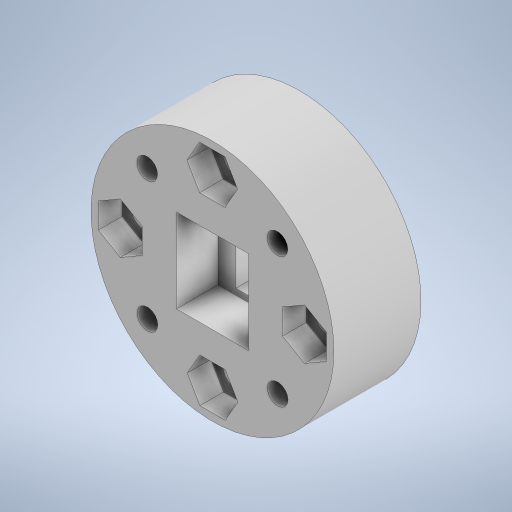
# Autodesk Inventor part: GripperBaseCircularLower
Saved by Autodesk Inventor 2023 (Build 270158000, 158)
## iProperties
Created: 2023-06-03
Part Number: GripperBaseCircularLower
Material: Ogólny
Document SubType Name: Modeling
Designer: Kamil
Density: 1 g/cm^3
Appearance: Domyślna
Author: Kamil
Autodesk Inventor part; units mm, degrees
ref_plane "YZ Plane" through (0, 0, 0) normal (1, 0, 0) x (0, 1, 0)
ref_plane "XZ Plane" through (0, 0, 0) normal (0, 1, 0) x (-1, 0, 0)
sketch "Szkic1" plane through (0, 0, 0) normal (0, 0, 1) x (1, 0, 0)
  line L0 (24.72, -24.72) -> (24.72, -14.42)
  line L1 (25.2197, -24.72) -> (24.72, -24.72)
  line L2 (24.72, -14.42) -> (25.2197, -14.42)
  line L3 (0, -39.14) -> (10.3, -39.14)
  line L4 (-14.42, -14.42) -> (-14.42, -24.72)
  line L5 (10.3, 0) -> (0, 0)
  line L6 (10.225, -25.645) -> (10.225, -13.495)
  line L7 (10.225, -25.645) -> (0.075, -25.645)
  line L8 (0.075, -13.495) -> (0.075, -25.645)
  line L9 (0.075, -13.495) -> (10.225, -13.495)
  line L10 (-14.9619, -24.72) -> (-14.9619, -24.7024)
  arc A0 (-14.9619, -24.7024) -> (0.075, -39.676) centre (5.1314, -19.5612) ccw
  arc A1 (10.3, -39.6475) -> (25.2201, -24.72) centre (5.1314, -19.5612) ccw
  line L11 (-14.9619, -14.42) -> (-14.42, -14.42)
  line L12 (24.72, -14.42) -> (25.2247, -14.42)
  line L13 (-14.42, -24.72) -> (-14.9619, -24.72)
  line L14 (0.075, -39.14) -> (0.075, -39.676)
  line L15 (0.075, 0.5536) -> (0.075, 0)
  line L16 (0.075, -13.495) -> (0.075, -25.645)
  line L17 (10.3, -39.6475) -> (10.3, -39.14)
  line L18 (10.3, 0) -> (10.3, 0.5251)
  line L19 (25.2201, -24.72) -> (24.72, -24.72)
  arc A2 (25.2247, -14.42) -> (10.3, 0.5251) centre (5.1314, -19.5612) ccw
  arc A3 (0.075, 0.5536) -> (-14.9619, -14.42) centre (5.1314, -19.5612) ccw
  circle A4 centre (5.1581, -35.1055) radius 1.75
  circle A5 centre (16.1418, -30.5337) radius 1.75
  circle A6 centre (20.6757, -19.5344) radius 1.75
  circle A7 centre (16.1039, -8.5508) radius 1.75
  circle A8 centre (5.1046, -4.0169) radius 1.75
  circle A9 centre (-5.879, -8.5887) radius 1.75
  circle A10 centre (-10.4129, -19.588) radius 1.75
  circle A11 centre (-5.8412, -30.5716) radius 1.75
  point P0 (5.15, -19.57)
  point P1 (-14.9574, -24.72)
  dimension "d0" = 3.5
  dimension "d3" = 360
  constraints: 40 end point, 12 centre point, 10 parallel, 8 point on circle, 2 horizontal, 2 point on line, 1 coincident, 17 other
  measures "d0" diameter of A4
extrude "Wyciągnięcie proste1" add sketch "Szkic1" along normal blind 9.7 contours L1 A1 L17 L3 L14 A0 L13 L4 L11 A3 L15 L5 L18 A2 L12 L2 L0
sketch "Szkic2" plane through (0, 0, 0) normal (0, 0, -1) x (-1, 0, 0)
  circle A0 centre (-16.1039, -8.5508) radius 1.75 projected
  circle A1 centre (-16.1039, -8.5508) radius 2.9
  arc A2 (-10.3, 0.5251) -> (-25.2247, -14.42) centre (-5.1314, -19.5612) ccw projected
  arc A3 (-0.075, -39.676) -> (14.9574, -24.72) centre (-5.1314, -19.5612) ccw projected
  circle A4 centre (-16.1418, -30.5337) radius 2.9
  circle A5 centre (5.8412, -30.5716) radius 2.9
  circle A6 centre (5.879, -8.5887) radius 2.9
  line L0 (-13.226, -10.2628) -> (-16.1476, -11.8991)
  line L1 (-16.1476, -11.8991) -> (-19.0255, -10.1871)
  line L2 (-19.0255, -10.1871) -> (-18.9818, -6.8387)
  line L3 (-18.9818, -6.8387) -> (-16.0602, -5.2024)
  line L4 (-16.0602, -5.2024) -> (-13.1823, -6.9145)
  line L5 (-13.1823, -6.9145) -> (-13.226, -10.2628)
  line L6 (-19.7668, -16.3115) -> (-17.4301, -18.71)
  line L7 (-23.0124, -17.1359) -> (-19.7668, -16.3115)
  line L8 (-23.9212, -20.3588) -> (-23.0124, -17.1359)
  line L9 (-21.5845, -22.7574) -> (-23.9212, -20.3588)
  line L10 (-18.3389, -21.933) -> (-21.5845, -22.7574)
  line L11 (-17.4301, -18.71) -> (-18.3389, -21.933)
  line L12 (-17.7781, -27.6121) -> (-14.4297, -27.6559)
  line L13 (-19.4901, -30.49) -> (-17.7781, -27.6121)
  line L14 (-17.8538, -33.4116) -> (-19.4901, -30.49)
  line L15 (-14.5055, -33.4554) -> (-17.8538, -33.4116)
  line L16 (-12.7934, -30.5775) -> (-14.5055, -33.4554)
  line L17 (-14.4297, -27.6559) -> (-12.7934, -30.5775)
  line L18 (-8.3811, -34.1966) -> (-5.9825, -31.8599)
  line L19 (-7.5567, -37.4422) -> (-8.3811, -34.1966)
  line L20 (-4.3338, -38.3511) -> (-7.5567, -37.4422)
  line L21 (-1.9352, -36.0143) -> (-4.3338, -38.3511)
  line L22 (-2.7596, -32.7688) -> (-1.9352, -36.0143)
  line L23 (-5.9825, -31.8599) -> (-2.7596, -32.7688)
  line L24 (2.9196, -32.2079) -> (2.9633, -28.8596)
  line L25 (5.7974, -33.92) -> (2.9196, -32.2079)
  line L26 (8.7191, -32.2837) -> (5.7974, -33.92)
  line L27 (8.7628, -28.9353) -> (8.7191, -32.2837)
  line L28 (5.8849, -27.2233) -> (8.7628, -28.9353)
  line L29 (2.9633, -28.8596) -> (5.8849, -27.2233)
  line L30 (9.5041, -22.8109) -> (7.1674, -20.4124)
  line L31 (12.7496, -21.9865) -> (9.5041, -22.8109)
  line L32 (13.6585, -18.7636) -> (12.7496, -21.9865)
  line L33 (11.3218, -16.365) -> (13.6585, -18.7636)
  line L34 (8.0762, -17.1894) -> (11.3218, -16.365)
  line L35 (7.1674, -20.4124) -> (8.0762, -17.1894)
  line L36 (7.5153, -11.5103) -> (4.167, -11.4666)
  line L37 (9.2274, -8.6324) -> (7.5153, -11.5103)
  line L38 (7.5911, -5.7108) -> (9.2274, -8.6324)
  line L39 (4.2427, -5.667) -> (7.5911, -5.7108)
  line L40 (2.5307, -8.5449) -> (4.2427, -5.667)
  line L41 (4.167, -11.4666) -> (2.5307, -8.5449)
  line L42 (-1.8817, -4.9258) -> (-4.2802, -7.2625)
  line L43 (-2.706, -1.6802) -> (-1.8817, -4.9258)
  line L44 (-5.929, -0.7713) -> (-2.706, -1.6802)
  line L45 (-8.3275, -3.1081) -> (-5.929, -0.7713)
  line L46 (-7.5031, -6.3536) -> (-8.3275, -3.1081)
  line L47 (-4.2802, -7.2625) -> (-7.5031, -6.3536)
  point P0 (0, 0)
  point P1 (-13.2042, -8.5887)
  point P2 (-18.5984, -17.5108)
  point P3 (-16.1039, -27.634)
  point P4 (-7.1818, -33.0283)
  point P5 (2.9414, -30.5337)
  point P6 (8.3357, -21.6116)
  point P7 (5.8412, -11.4884)
  point P8 (-3.0809, -6.0941)
  dimension "d7" = 5.8
  dimension "d10" = 360
  dimension "d22" = 360
  constraints: 96 end point, 3 centre point, 2 coincident, 1 midpoint, 130 other
extrude "Wyciągnięcie proste2" cut sketch "Szkic2" against normal blind 3.7 contours A1 | A4 | A5 | A6
sketch "Szkic3" plane through (0, 0, 0) normal (0, 0, -1) x (-1, 0, 0)
  circle A0 centre (5.8412, -30.5716) radius 2.9 projected
  circle A1 centre (5.879, -8.5887) radius 2.9 projected
  circle A2 centre (-16.1418, -30.5337) radius 2.9 projected
  circle A3 centre (-16.1039, -8.5508) radius 2.9 projected
  line L0 (-24.72, -14.42) -> (-25.2247, -14.42) projected
  line L1 (-24.72, -24.72) -> (-24.72, -14.42) projected
  line L2 (-25.2201, -24.72) -> (-24.72, -24.72) projected
  arc A4 (-25.2201, -24.72) -> (-10.3, -39.6475) centre (-5.1314, -19.5612) ccw projected
  line L3 (-10.3, -39.14) -> (-10.3, -39.6475) projected
  line L4 (-0.075, -39.14) -> (-10.3, -39.14) projected
  line L5 (-0.075, -39.676) -> (-0.075, -39.14) projected
  arc A5 (-0.075, -39.676) -> (14.9574, -24.72) centre (-5.1314, -19.5612) ccw projected
  line L6 (14.42, -24.72) -> (14.9574, -24.72) projected
  line L7 (14.42, -14.42) -> (14.42, -24.72) projected
  line L8 (14.9619, -14.42) -> (14.42, -14.42) projected
  arc A6 (14.9619, -14.42) -> (-0.075, 0.5536) centre (-5.1314, -19.5612) ccw projected
  line L9 (-0.075, 0) -> (-0.075, 0.5536) projected
  line L10 (-10.3, 0) -> (-0.075, 0) projected
  line L11 (-10.3, 0.5251) -> (-10.3, 0) projected
  arc A7 (-10.3, 0.5251) -> (-25.2247, -14.42) centre (-5.1314, -19.5612) ccw projected
  circle A8 centre (10.4129, -19.588) radius 1.75 projected
  circle A9 centre (-5.1581, -35.1055) radius 1.75 projected
  circle A10 centre (-20.6757, -19.5344) radius 1.75 projected
  circle A11 centre (-5.1046, -4.0169) radius 1.75 projected
  line L12 (-10.225, -25.645) -> (-0.075, -25.645) projected
  line L13 (-10.225, -13.495) -> (-10.225, -25.645) projected
  line L14 (-0.075, -13.495) -> (-10.225, -13.495) projected
  line L15 (-0.075, -25.645) -> (-0.075, -13.495) projected
  line L16 (-10.225, -13.495) -> (-8.225, -13.495)
  line L17 (-8.225, -13.495) -> (-8.225, -25.645)
  line L18 (-8.225, -25.645) -> (-10.225, -25.645)
  line L19 (-10.225, -25.645) -> (-10.225, -13.495)
  line L20 (-0.075, -25.645) -> (-2.075, -25.645)
  line L21 (-2.075, -25.645) -> (-2.075, -13.495)
  line L22 (-2.075, -13.495) -> (-0.075, -13.495)
  line L23 (-0.075, -13.495) -> (-0.075, -25.645)
  point P0 (0, 0)
  dimension "d14" = 2
  dimension "d15" = 2
  constraints: 16 end point, 4 parallel, 2 horizontal, 2 perpendicular, 2 point on line
  measures "d14" distance of L17.end L18.end
  measures "d15" distance of L21.end L22.end
extrude "Wyciągnięcie proste3" add sketch "Szkic3" against normal blind 4.7 contours L13 L14 L17 L12 | L21 L14 L15 L12
sketch "Szkic4" plane through (0, 0, 9.7) normal (0, 0, 1) x (1, 0, 0)
  line L0 (24.72, -14.42) -> (25.2247, -14.42) projected
  arc A0 (25.2247, -14.42) -> (10.3, 0.5251) centre (5.1314, -19.5612) ccw projected
  line L1 (10.3, 0.5251) -> (10.3, 0) projected
  line L2 (10.3, 0) -> (0.075, 0) projected
  line L3 (0.075, 0) -> (0.075, 0.5536) projected
  arc A1 (0.075, 0.5536) -> (-14.9619, -14.42) centre (5.1314, -19.5612) ccw projected
  line L4 (-14.9619, -14.42) -> (-14.42, -14.42) projected
  line L5 (-14.42, -14.42) -> (-14.42, -24.72) projected
  line L6 (-14.42, -24.72) -> (-14.9574, -24.72) projected
  arc A2 (-14.9574, -24.72) -> (0.075, -39.676) centre (5.1314, -19.5612) ccw projected
  line L7 (0.075, -39.676) -> (0.075, -39.14) projected
  line L8 (0.075, -39.14) -> (10.3, -39.14) projected
  line L9 (10.3, -39.14) -> (10.3, -39.6475) projected
  arc A3 (10.3, -39.6475) -> (25.2201, -24.72) centre (5.1314, -19.5612) ccw projected
  line L10 (25.2201, -24.72) -> (24.72, -24.72) projected
  line L11 (24.72, -24.72) -> (24.72, -14.42) projected
  circle A4 centre (-10.4129, -19.588) radius 1.75 projected
  circle A5 centre (5.1581, -35.1055) radius 1.75 projected
  circle A6 centre (20.6757, -19.5344) radius 1.75 projected
  circle A7 centre (5.1046, -4.0169) radius 1.75 projected
  circle A8 centre (-5.8412, -30.5716) radius 1.75 projected
  circle A9 centre (-5.879, -8.5887) radius 1.75 projected
  circle A10 centre (16.1039, -8.5508) radius 1.75 projected
  circle A11 centre (16.1418, -30.5337) radius 1.75 projected
  line L12 (10.225, -25.645) -> (0.075, -25.645) projected
  line L13 (0.075, -25.645) -> (0.075, -13.495) projected
  line L14 (0.075, -13.495) -> (10.225, -13.495) projected
  line L15 (10.225, -13.495) -> (10.225, -25.645) projected
  line L16 (10.3, 0.5251) -> (10.3, 0) projected
  line L17 (10.3, 0.5251) -> (0.075, 0.5536)
  line L18 (10.3, 0) -> (0.075, 0) projected
  circle A12 centre (5.1314, -19.5612) radius 20.2325
  point P0 (0, 0)
  point P1 (-14.4371, -14.42)
  point P2 (0.075, 0.0293)
  point P3 (0.075, -39.1517)
  point P4 (-14.4324, -24.72)
  point P5 (24.72, -24.6249)
  point P6 (10.2329, -39.14)
  point P7 (24.72, -14.4975)
  constraints: 2 end point, 1 coincident, 3 other
extrude "Wyciągnięcie proste4" cut sketch "Szkic4" against normal through all contours L11 A12 L1 A0 L0 | L11 L10 A3 L9 L8 A12 | L7 A2 L6 A12 | A12 L4 A1 L3
sketch "Szkic5" plane through (0, 0, 0) normal (0, 0, -1) x (-1, 0, 0)
  circle A0 centre (-16.1039, -8.5508) radius 2.9 projected
  circle A1 centre (-16.1039, -8.5508) radius 2.9 projected
  line L0 (-13.2039, -10.2251) -> (-16.1039, -11.8994)
  line L1 (-16.1039, -11.8994) -> (-19.0039, -10.2251)
  line L2 (-19.0039, -10.2251) -> (-19.0039, -6.8765)
  line L3 (-19.0039, -6.8765) -> (-16.1039, -5.2022)
  line L4 (-16.1039, -5.2022) -> (-13.2039, -6.8765)
  line L5 (-13.2039, -6.8765) -> (-13.2039, -10.2251)
  arc A2 (-10.3, 0) -> (-24.72, -14.4975) centre (-5.1314, -19.5612) ccw projected
  line L6 (-17.4411, -18.6677) -> (-18.3078, -21.9023)
  line L7 (-18.3078, -21.9023) -> (-21.5423, -22.769)
  line L8 (-21.5423, -22.769) -> (-23.9102, -20.4011)
  line L9 (-23.9102, -20.4011) -> (-23.0435, -17.1666)
  line L10 (-23.0435, -17.1666) -> (-19.809, -16.2999)
  line L11 (-19.809, -16.2999) -> (-17.4411, -18.6677)
  line L12 (-14.4675, -27.6337) -> (-12.7931, -30.5337)
  line L13 (-12.7931, -30.5337) -> (-14.4675, -33.4337)
  line L14 (-14.4675, -33.4337) -> (-17.8161, -33.4337)
  line L15 (-17.8161, -33.4337) -> (-19.4904, -30.5337)
  line L16 (-19.4904, -30.5337) -> (-17.8161, -27.6337)
  line L17 (-17.8161, -27.6337) -> (-14.4675, -27.6337)
  line L18 (-6.0248, -31.871) -> (-2.7903, -32.7377)
  line L19 (-2.7903, -32.7377) -> (-1.9236, -35.9722)
  line L20 (-1.9236, -35.9722) -> (-4.2915, -38.34)
  line L21 (-4.2915, -38.34) -> (-7.526, -37.4733)
  line L22 (-7.526, -37.4733) -> (-8.3927, -34.2388)
  line L23 (-8.3927, -34.2388) -> (-6.0248, -31.871)
  line L24 (2.9412, -28.8973) -> (5.8412, -27.223)
  line L25 (5.8412, -27.223) -> (8.7412, -28.8973)
  line L26 (8.7412, -28.8973) -> (8.7412, -32.2459)
  line L27 (8.7412, -32.2459) -> (5.8412, -33.9202)
  line L28 (5.8412, -33.9202) -> (2.9412, -32.2459)
  line L29 (2.9412, -32.2459) -> (2.9412, -28.8973)
  line L30 (7.1784, -20.4547) -> (8.0451, -17.2201)
  line L31 (8.0451, -17.2201) -> (11.2796, -16.3534)
  line L32 (11.2796, -16.3534) -> (13.6475, -18.7213)
  line L33 (13.6475, -18.7213) -> (12.7808, -21.9558)
  line L34 (12.7808, -21.9558) -> (9.5462, -22.8225)
  line L35 (9.5462, -22.8225) -> (7.1784, -20.4547)
  line L36 (4.2047, -11.4887) -> (2.5304, -8.5887)
  line L37 (2.5304, -8.5887) -> (4.2047, -5.6887)
  line L38 (4.2047, -5.6887) -> (7.5534, -5.6887)
  line L39 (7.5534, -5.6887) -> (9.2277, -8.5887)
  line L40 (9.2277, -8.5887) -> (7.5534, -11.4887)
  line L41 (7.5534, -11.4887) -> (4.2047, -11.4887)
  line L42 (-4.2379, -7.2514) -> (-7.4724, -6.3847)
  line L43 (-7.4724, -6.3847) -> (-8.3391, -3.1502)
  line L44 (-8.3391, -3.1502) -> (-5.9713, -0.7824)
  line L45 (-5.9713, -0.7824) -> (-2.7367, -1.6491)
  line L46 (-2.7367, -1.6491) -> (-1.8701, -4.8836)
  line L47 (-1.8701, -4.8836) -> (-4.2379, -7.2514)
  point P0 (0, 0)
  point P1 (-13.2039, -8.5508)
  point P2 (-20.6757, -19.5344)
  point P3 (-18.625, -17.4838)
  point P4 (-16.1418, -30.5337)
  point P5 (-16.1418, -27.6337)
  point P6 (-5.1581, -35.1055)
  point P7 (-7.2088, -33.0549)
  point P8 (5.8412, -30.5716)
  point P9 (2.9412, -30.5716)
  point P10 (10.4129, -19.588)
  point P11 (8.3623, -21.6386)
  point P12 (5.879, -8.5887)
  point P13 (5.879, -11.4887)
  point P14 (-5.1046, -4.0169)
  point P15 (-3.054, -6.0675)
  dimension "d26" = 360
  constraints: 96 end point, 1 coincident, 1 horizontal alignment, 1 midpoint, 127 other
extrude "Wyciągnięcie proste5" cut sketch "Szkic5" against normal blind 4 contours A0 | L5 L0 A0 | A0 L4 L5 | A0 L3 L4 | L0 L1 A0 | A0 L2 L3 | L1 L2 A0 | L12 L13 L14 L15 L16 L17 | L24 L25 L26 L27 L28 L29 | L36 L37 L38 L39 L40 L41
sketch "Szkic6" plane through (0, 0, 9.7) normal (0, 0, 1) x (1, 0, 0)
  line L0 (10.225, -25.645) -> (0.075, -25.645) projected
  line L1 (0.075, -25.645) -> (0.075, -13.495) projected
  line L2 (0.075, -13.495) -> (10.225, -13.495) projected
  line L3 (10.225, -13.495) -> (10.225, -25.645) projected
  circle A0 centre (16.1418, -30.5337) radius 1.75 projected
  circle A1 centre (16.1039, -8.5508) radius 1.75 projected
  circle A2 centre (-5.879, -8.5887) radius 1.75 projected
  circle A3 centre (-5.8412, -30.5716) radius 1.75 projected
  circle A4 centre (5.1046, -4.0169) radius 1.75 projected
  circle A5 centre (20.6757, -19.5344) radius 1.75 projected
  circle A6 centre (5.1581, -35.1055) radius 1.75 projected
  circle A7 centre (-10.4129, -19.588) radius 1.75 projected
  arc A8 (-14.4324, -24.72) -> (0.075, -39.1517) centre (5.1314, -19.5612) ccw projected
  line L4 (0.075, -39.1517) -> (0.075, -39.14) projected
  line L5 (0.075, -39.14) -> (10.2329, -39.14) projected
  arc A9 (10.2329, -39.14) -> (24.72, -24.6249) centre (5.1314, -19.5612) ccw projected
  line L6 (24.72, -24.6249) -> (24.72, -14.4975) projected
  arc A10 (24.72, -14.4975) -> (10.3, 0) centre (5.1314, -19.5612) ccw projected
  line L7 (10.3, 0) -> (0.075, 0) projected
  line L8 (0.075, 0) -> (0.075, 0.0293) projected
  arc A11 (0.075, 0.0293) -> (-14.4371, -14.42) centre (5.1314, -19.5612) ccw projected
  line L9 (-14.4371, -14.42) -> (-14.42, -14.42) projected
  line L10 (-14.42, -14.42) -> (-14.42, -24.72) projected
  line L11 (-14.42, -24.72) -> (-14.4324, -24.72) projected
  circle A12 centre (5.1046, -4.0169) radius 1.75 projected
  circle A13 centre (5.1046, -4.0169) radius 2.25
  circle A14 centre (-10.4129, -19.588) radius 1.75 projected
  circle A15 centre (-10.4129, -19.588) radius 2.25
  circle A16 centre (5.1581, -35.1055) radius 1.75 projected
  circle A17 centre (5.1581, -35.1055) radius 2.25
  circle A18 centre (20.6757, -19.5344) radius 2.25
  point P0 (0, 0)
  dimension "d30" = 4.5
  dimension "d31" = 4.5
  dimension "d32" = 4.5
  dimension "d33" = 4.5
  constraints: 4 centre point, 4 coincident
  measures "d30" diameter of A13
  measures "d31" diameter of A15
  measures "d32" diameter of A17
  measures "d33" diameter of A18
extrude "Wyciągnięcie proste6" cut sketch "Szkic6" against normal through all contours A4 | A5 | A6 | A7 | A13 | A15 | A17 | A18
sketch "Szkic7" plane through (0, 0, 9.7) normal (0, 0, 1) x (1, 0, 0)
  circle A0 centre (5.1581, -35.1055) radius 2.25 projected
  circle A1 centre (-10.4129, -19.588) radius 2.25 projected
  circle A2 centre (20.6757, -19.5344) radius 2.25 projected
  circle A3 centre (5.1046, -4.0169) radius 2.25 projected
  line L0 (10.225, -25.645) -> (0.075, -25.645) projected
  line L1 (0.075, -25.645) -> (0.075, -13.495) projected
  line L2 (0.075, -13.495) -> (10.225, -13.495) projected
  line L3 (10.225, -13.495) -> (10.225, -25.645) projected
  circle A4 centre (16.1418, -30.5337) radius 1.75 projected
  circle A5 centre (16.1039, -8.5508) radius 1.75 projected
  circle A6 centre (-5.879, -8.5887) radius 1.75 projected
  circle A7 centre (-5.8412, -30.5716) radius 1.75 projected
  arc A8 (-14.4324, -24.72) -> (0.075, -39.1517) centre (5.1314, -19.5612) ccw projected
  line L4 (0.075, -39.1517) -> (0.075, -39.14) projected
  line L5 (0.075, -39.14) -> (10.2329, -39.14) projected
  arc A9 (10.2329, -39.14) -> (24.72, -24.6249) centre (5.1314, -19.5612) ccw projected
  line L6 (24.72, -24.6249) -> (24.72, -14.4975) projected
  arc A10 (24.72, -14.4975) -> (10.3, 0) centre (5.1314, -19.5612) ccw projected
  line L7 (10.3, 0) -> (0.075, 0) projected
  line L8 (0.075, 0) -> (0.075, 0.0293) projected
  arc A11 (0.075, 0.0293) -> (-14.4371, -14.42) centre (5.1314, -19.5612) ccw projected
  line L9 (-14.4371, -14.42) -> (-14.42, -14.42) projected
  line L10 (-14.42, -14.42) -> (-14.42, -24.72) projected
  line L11 (-14.42, -24.72) -> (-14.4324, -24.72) projected
  line L12 (-14.2545, -13.7696) -> (-14.6283, -14.1018)
  circle A12 centre (5.1314, -19.5612) radius 20.5
  point P0 (0, 0)
  dimension "d46" = 41
  dimension "d36" = 0.5
  constraints: 2 end point, 1 coincident, 1 point on circle, 3 other
  measures "d36" distance of L12.start L12.end
extrude "Wyciągnięcie proste7" add sketch "Szkic7" against normal up to surface (9.7 mm away) contours A12
sketch "Szkic8" plane through (5.1314, -19.5612, 9.7) normal (0, 0, 1) x (1, 0, 0)
  circle A0 centre (0, 0) radius 20.5 projected
  circle A1 centre (0.0268, -15.5443) radius 2.25 projected
  circle A2 centre (-15.5443, -0.0268) radius 2.25 projected
  circle A3 centre (15.5443, 0.0268) radius 2.25 projected
  circle A4 centre (-0.0268, 15.5443) radius 2.25 projected
  line L0 (5.0936, -6.0838) -> (-5.0564, -6.0838) projected
  line L1 (-5.0564, -6.0838) -> (-5.0564, 6.0662) projected
  line L2 (-5.0564, 6.0662) -> (5.0936, 6.0662) projected
  line L3 (5.0936, 6.0662) -> (5.0936, -6.0838) projected
  circle A5 centre (11.0104, -10.9725) radius 1.75 projected
  circle A6 centre (10.9725, 11.0104) radius 1.75 projected
  circle A7 centre (-11.0104, 10.9725) radius 1.75 projected
  circle A8 centre (-10.9725, -11.0104) radius 1.75 projected
  circle A9 centre (-0.0268, 15.5443) radius 3.7
  circle A10 centre (-0.0268, 15.5443) radius 2.25 projected
  line L4 (2.1094, 19.2443) -> (4.2456, 15.5443)
  line L5 (4.2456, 15.5443) -> (2.1094, 11.8443)
  line L6 (2.1094, 11.8443) -> (-2.163, 11.8443)
  line L7 (-2.163, 11.8443) -> (-4.2992, 15.5443)
  line L8 (-4.2992, 15.5443) -> (-2.163, 19.2443)
  line L9 (-2.163, 19.2443) -> (2.1094, 19.2443)
  line L10 (-6.8836, 9.8668) -> (-9.9046, 6.8457)
  line L11 (-7.9894, 13.9936) -> (-6.8836, 9.8668)
  line L12 (-9.9046, 6.8457) -> (-14.0314, 7.9515)
  line L13 (-12.1162, 15.0994) -> (-7.9894, 13.9936)
  line L14 (-15.1372, 12.0783) -> (-12.1162, 15.0994)
  circle A11 centre (-11.0104, 10.9725) radius 3.7
  line L15 (-14.0314, 7.9515) -> (-15.1372, 12.0783)
  line L16 (-11.8443, 2.1094) -> (-11.8443, -2.163)
  line L17 (-15.5443, 4.2456) -> (-11.8443, 2.1094)
  line L18 (-11.8443, -2.163) -> (-15.5443, -4.2992)
  line L19 (-19.2443, 2.1094) -> (-15.5443, 4.2456)
  line L20 (-19.2443, -2.163) -> (-19.2443, 2.1094)
  circle A12 centre (-15.5443, -0.0268) radius 3.7
  line L21 (-15.5443, -4.2992) -> (-19.2443, -2.163)
  line L22 (-9.8668, -6.8836) -> (-6.8457, -9.9046)
  line L23 (-13.9936, -7.9894) -> (-9.8668, -6.8836)
  line L24 (-6.8457, -9.9046) -> (-7.9515, -14.0314)
  line L25 (-15.0994, -12.1162) -> (-13.9936, -7.9894)
  line L26 (-12.0783, -15.1372) -> (-15.0994, -12.1162)
  circle A13 centre (-10.9725, -11.0104) radius 3.7
  line L27 (-7.9515, -14.0314) -> (-12.0783, -15.1372)
  line L28 (-2.1094, -11.8443) -> (2.163, -11.8443)
  line L29 (-4.2456, -15.5443) -> (-2.1094, -11.8443)
  line L30 (2.163, -11.8443) -> (4.2992, -15.5443)
  line L31 (-2.1094, -19.2443) -> (-4.2456, -15.5443)
  line L32 (2.163, -19.2443) -> (-2.1094, -19.2443)
  circle A14 centre (0.0268, -15.5443) radius 3.7
  line L33 (4.2992, -15.5443) -> (2.163, -19.2443)
  line L34 (6.8836, -9.8668) -> (9.9046, -6.8457)
  line L35 (7.9894, -13.9936) -> (6.8836, -9.8668)
  line L36 (9.9046, -6.8457) -> (14.0314, -7.9515)
  line L37 (12.1162, -15.0994) -> (7.9894, -13.9936)
  line L38 (15.1372, -12.0783) -> (12.1162, -15.0994)
  circle A15 centre (11.0104, -10.9725) radius 3.7
  line L39 (14.0314, -7.9515) -> (15.1372, -12.0783)
  line L40 (11.8443, -2.1094) -> (11.8443, 2.163)
  line L41 (15.5443, -4.2456) -> (11.8443, -2.1094)
  line L42 (11.8443, 2.163) -> (15.5443, 4.2992)
  line L43 (19.2443, -2.1094) -> (15.5443, -4.2456)
  line L44 (19.2443, 2.163) -> (19.2443, -2.1094)
  circle A16 centre (15.5443, 0.0268) radius 3.7
  line L45 (15.5443, 4.2992) -> (19.2443, 2.163)
  line L46 (9.8668, 6.8836) -> (6.8457, 9.9046)
  line L47 (13.9936, 7.9894) -> (9.8668, 6.8836)
  line L48 (6.8457, 9.9046) -> (7.9515, 14.0314)
  line L49 (15.0994, 12.1162) -> (13.9936, 7.9894)
  line L50 (12.0783, 15.1372) -> (15.0994, 12.1162)
  circle A17 centre (10.9725, 11.0104) radius 3.7
  line L51 (7.9515, 14.0314) -> (12.0783, 15.1372)
  point P0 (-5.1314, 19.5612)
  point P1 (-0.0268, 19.2443)
  point P2 (-13.6267, 13.5888)
  point P3 (-19.2443, -0.0268)
  point P4 (-13.5888, -13.6267)
  point P5 (0.0268, -19.2443)
  point P6 (13.6267, -13.5888)
  point P7 (19.2443, 0.0268)
  point P8 (13.5888, 13.6267)
  dimension "d39" = 7.4
  dimension "d42" = 360
  constraints: 96 end point, 2 coincident, 2 horizontal alignment, 2 vertical alignment, 1 midpoint, 162 other
extrude "Wyciągnięcie proste8" cut sketch "Szkic8" against normal blind 4 contours A1 | A2 | A3 | A4 | A9 | A9 L4 L5 | A9 L9 L4 | L5 L6 A9 | A9 L8 L9 | L6 L7 A9 | A9 L7 L8 | L16 A12 L17 | A12 | L16 L18 A12 | A12 L19 L17 | L18 L21 A12 | A12 L20 L19 | L21 L20 A12 | L28 A14 L29 | L28 L30 A14 | A14 | A14 L31 L29 | L30 L33 A14 | A14 L32 L31 | A14 L33 L32 | L40 A16 L41 | L40 L42 A16 | A16 | A16 L43 L41 | L42 L45 A16 | A16 L44 L43 | L45 L44 A16
ref_plane "Płaszczyzna konstrukcyjna1" through (0, 0, 4.85) normal (0, 0, -1) x (-1, 0, 0)
sketch "Szkic9" plane through (5.1314, -19.5612, 0) normal (0, 0, -1) x (-1, 0, 0)
  circle A0 centre (0, 0) radius 20.5 projected
  circle A1 centre (-0.0268, -15.5443) radius 2.25 projected
  circle A2 centre (15.5443, -0.0268) radius 2.25 projected
  circle A3 centre (-15.5443, 0.0268) radius 2.25 projected
  circle A4 centre (0.0268, 15.5443) radius 2.25 projected
  line L0 (10.9725, -14.359) -> (8.0725, -12.6847) projected
  line L1 (8.0725, -12.6847) -> (8.0725, -9.3361) projected
  line L2 (8.0725, -9.3361) -> (10.9725, -7.6618) projected
  line L3 (10.9725, -7.6618) -> (13.8725, -9.3361) projected
  line L4 (13.8725, -9.3361) -> (13.8725, -12.6847) projected
  line L5 (13.8725, -12.6847) -> (10.9725, -14.359) projected
  line L6 (14.359, 10.9725) -> (12.6847, 8.0725) projected
  line L7 (12.6847, 8.0725) -> (9.3361, 8.0725) projected
  line L8 (9.3361, 8.0725) -> (7.6618, 10.9725) projected
  line L9 (7.6618, 10.9725) -> (9.3361, 13.8725) projected
  line L10 (9.3361, 13.8725) -> (12.6847, 13.8725) projected
  line L11 (12.6847, 13.8725) -> (14.359, 10.9725) projected
  line L12 (-14.359, -10.9725) -> (-12.6847, -8.0725) projected
  line L13 (-12.6847, -8.0725) -> (-9.3361, -8.0725) projected
  line L14 (-9.3361, -8.0725) -> (-7.6618, -10.9725) projected
  line L15 (-7.6618, -10.9725) -> (-9.3361, -13.8725) projected
  line L16 (-9.3361, -13.8725) -> (-12.6847, -13.8725) projected
  line L17 (-12.6847, -13.8725) -> (-14.359, -10.9725) projected
  line L18 (-10.9725, 14.359) -> (-8.0725, 12.6847) projected
  line L19 (-8.0725, 12.6847) -> (-8.0725, 9.3361) projected
  line L20 (-8.0725, 9.3361) -> (-10.9725, 7.6618) projected
  line L21 (-10.9725, 7.6618) -> (-13.8725, 9.3361) projected
  line L22 (-13.8725, 9.3361) -> (-13.8725, 12.6847) projected
  line L23 (-13.8725, 12.6847) -> (-10.9725, 14.359) projected
  line L24 (-3.0936, -6.0838) -> (-3.0936, 6.0662) projected
  line L25 (3.0564, 6.0662) -> (-3.0936, 6.0662) projected
  line L26 (3.0564, 6.0662) -> (3.0564, -6.0838) projected
  line L27 (-3.0936, -6.0838) -> (3.0564, -6.0838) projected
  line L28 (3.0564, -6.0838) -> (8.7659, -5.9818) construction
  circle A5 centre (0, 0) radius 20.5 projected
  line L29 (8.7659, -5.9818) -> (18.4857, -8.8616) construction
  spline S0 degree 2 poles (3.0564, -6.0838) (8.7659, -5.9818) (18.4857, -8.8616) knots 1 1 1 2 2 2
  line L30 (3.0564, 6.0662) -> (8.0725, -1.5295) construction
  line L31 (8.0725, -1.5295) -> (20, -5) construction
  spline S1 degree 2 poles (3.0564, 6.0662) (8.0725, -1.5295) (20, -5) knots 1 1 1 2 2 2
  point P0 (5.1314, 19.5612)
  point P1 (18.4857, -8.8616)
  point P2 (19.889, -4.9676)
  constraints: 8 other
extrude "Wyciągnięcie proste9" cut sketch "Szkic9" against normal up to surface (4.85 mm away) contours S0 L26 S1 A0
fillet "Zaokrąglenie1" radius 4 2 edges at (-13.3544, -28.4228, 2.425) (-14.7577, -24.5288, 2.425)
fillet "Zaokrąglenie5" radius 1 1 edges at (2.075, -13.495, 2.35)
sketch "Szkic11" plane through (0, 0, 0) normal (0, 0, -1) x (-1, 0, 0)
  spline S0 degree 6 poles (15.3601, -18.9713) (15.3655, -19.1569) (15.3606, -19.3459) (15.3448, -19.5373) (15.3175, -19.7301) (15.2784, -19.9231) (15.1924, -20.2463) (15.1519, -20.3769) (15.1057, -20.5068) (15.0539, -20.6353) (14.9965, -20.7623) (14.8894, -20.9747) (14.8425, -21.0612) (14.793, -21.1466) (14.7408, -21.2308) (14.6859, -21.3135) (14.4924, -21.5874) (14.3418, -21.7716) (14.1776, -21.9455) (14.0009, -22.1075) (13.8129, -22.2565) (13.4176, -22.526) (13.2103, -22.6466) (12.9949, -22.7519) (12.7731, -22.8412) (12.5466, -22.9142) (12.2209, -22.9943) (12.1239, -23.0151) (12.0265, -23.033) (11.9289, -23.0479) (11.8312, -23.06) (11.5944, -23.0821) (11.4552, -23.0892) (11.3166, -23.0904) (11.1789, -23.086) (11.0425, -23.0759) (10.7102, -23.038) (10.5163, -23.0039) (10.3268, -22.9589) (10.1428, -22.9037) (9.9651, -22.8392) (9.7943, -22.7665) knots 0 0 0 0 0 0 0 0.151603 0.151603 0.151603 0.151603 0.151603 0.255165 0.255165 0.255165 0.255165 0.255165 0.32775 0.32775 0.32775 0.32775 0.32775 0.5 0.5 0.5 0.5 0.5 0.67225 0.67225 0.67225 0.67225 0.67225 0.744835 0.744835 0.744835 0.744835 0.744835 0.848397 0.848397 0.848397 0.848397 0.848397 1 1 1 1 1 1 1 projected
  arc A0 (15.3601, -18.9713) -> (9.8275, -33.5784) centre (-5.1314, -19.5612) ccw projected
  spline S1 degree 6 poles (7.8131, -26.9469) (8.1547, -27.0262) (8.4879, -27.1414) (8.8081, -27.2915) (9.1107, -27.4745) (9.3916, -27.6877) (9.9017, -28.1668) (10.1313, -28.4327) (10.3322, -28.7218) (10.5018, -29.0305) (10.6376, -29.3544) (10.8393, -30.0232) (10.905, -30.3682) (10.9344, -30.7191) (10.9267, -31.0712) (10.8824, -31.4196) (10.7227, -32.0982) (10.6077, -32.4285) (10.4584, -32.7459) (10.2767, -33.0459) (10.0654, -33.3246) (9.8275, -33.5784) knots 0 0 0 0 0 0 0 0.251 0.251 0.251 0.251 0.251 0.501 0.501 0.501 0.501 0.501 0.751 0.751 0.751 0.751 0.751 1 1 1 1 1 1 1 projected
  spline S2 degree 2 poles (7.8131, -26.9469) (1.8981, -25.574) (-2.075, -25.645) knots 0 0 0 1 1 1 projected
  line L0 (-8.225, -25.645) -> (-2.075, -25.645) projected
  line L1 (-8.225, -25.645) -> (-8.225, -13.495) projected
  line L2 (-2.6048, -13.495) -> (-8.225, -13.495) projected
  spline S3 degree 2 poles (-1.7844, -13.9232) (-2.0829, -13.495) (-2.6048, -13.495) knots 0 0 0 1 1 1 weights 1 0.886512 1 projected
  spline S4 degree 2 poles (-1.7844, -13.9232) (2.0929, -19.4861) (9.7943, -22.7665) knots 0 0 0 1 1 1 projected
  line L3 (-16.1039, -5.2022) -> (-13.2039, -6.8765) projected
  line L4 (-13.2039, -6.8765) -> (-13.2039, -10.2251) projected
  line L5 (-13.2039, -10.2251) -> (-16.1039, -11.8994) projected
  line L6 (-16.1039, -11.8994) -> (-19.0039, -10.2251) projected
  line L7 (-19.0039, -10.2251) -> (-19.0039, -6.8765) projected
  line L8 (-19.0039, -6.8765) -> (-16.1039, -5.2022) projected
  line L9 (-19.4904, -30.5337) -> (-17.8161, -27.6337) projected
  line L10 (-17.8161, -27.6337) -> (-14.4675, -27.6337) projected
  line L11 (-14.4675, -27.6337) -> (-12.7931, -30.5337) projected
  line L12 (-12.7931, -30.5337) -> (-14.4675, -33.4337) projected
  line L13 (-14.4675, -33.4337) -> (-17.8161, -33.4337) projected
  line L14 (-17.8161, -33.4337) -> (-19.4904, -30.5337) projected
  line L15 (9.2277, -8.5887) -> (7.5534, -11.4887) projected
  line L16 (7.5534, -11.4887) -> (4.2047, -11.4887) projected
  line L17 (4.2047, -11.4887) -> (2.5304, -8.5887) projected
  line L18 (2.5304, -8.5887) -> (4.2047, -5.6887) projected
  line L19 (4.2047, -5.6887) -> (7.5534, -5.6887) projected
  line L20 (7.5534, -5.6887) -> (9.2277, -8.5887) projected
  line L21 (5.8412, -33.9202) -> (2.9412, -32.2459) projected
  line L22 (2.9412, -32.2459) -> (2.9412, -28.8973) projected
  line L23 (2.9412, -28.8973) -> (5.8412, -27.223) projected
  line L24 (5.8412, -27.223) -> (8.7412, -28.8973) projected
  line L25 (8.7412, -28.8973) -> (8.7412, -32.2459) projected
  line L26 (8.7412, -32.2459) -> (5.8412, -33.9202) projected
  circle A1 centre (-5.1046, -4.0169) radius 2.25 projected
  circle A2 centre (-20.6757, -19.5344) radius 2.25 projected
  circle A3 centre (10.4129, -19.588) radius 2.25 projected
  circle A4 centre (-5.1581, -35.1055) radius 2.25 projected
  point P0 (0, 0)
  constraints: 5 other
extrude "Wyciągnięcie proste11" add sketch "Szkic11" along normal blind 5
fillet "Zaokrąglenie6" radius 1 1 edges at (0.075, -20.8541, 4.85)
sketch "Szkic12" plane through (5.1314, -19.5612, 9.7) normal (0, 0, 1) x (1, 0, 0)
  line L0 (5.0936, 6.0662) -> (5.0936, -6.0838) projected
  line L1 (-5.0564, 6.0662) -> (5.0936, 6.0662) projected
  line L2 (-5.0564, -6.0838) -> (-5.0564, 6.0662) projected
  line L3 (5.0936, -6.0838) -> (-5.0564, -6.0838) projected
  line L4 (6.0936, -7.0838) -> (6.0936, 7.0662)
  line L5 (6.0936, 7.0662) -> (-6.0564, 7.0662)
  line L6 (-6.0564, 7.0662) -> (-6.0564, -7.0838)
  line L7 (-6.0564, -7.0838) -> (6.0936, -7.0838)
  point P0 (-5.1314, 19.5612)
  dimension "d59" = 1
  constraints: 8 end point, 3 other
  measures "d59" distance between parallel lines of L0 L4
extrude "Wyciągnięcie proste12" cut sketch "Szkic12" against normal up to surface (5 mm away)
sketch "Szkic13" plane through (0, 0, 4.7) normal (0, 0, 1) x (1, 0, 0)
  line L0 (2.075, -25.645) -> (8.225, -25.645) projected
  spline S0 degree 4 poles (2.075, -25.645) (1.8972, -25.6418) (1.7193, -25.6406) (1.5414, -25.6413) (1.3414, -25.6439) (1.3192, -25.6443) (1.2971, -25.6446) (1.2749, -25.645) knots 0 0 0 0 0 0.889259 0.889259 0.889259 1 1 1 1 1 projected
  spline S1 degree 6 poles (-0.925, -25.7704) (-0.5591, -25.7365) (-0.1928, -25.7072) (0.1738, -25.6829) (0.5407, -25.6641) (0.9078, -25.6513) (1.2749, -25.645) knots 0 0 0 0 0 0 0 1 1 1 1 1 1 1 projected
  line L1 (-0.925, -26.645) -> (-0.925, -25.7704) projected
  line L2 (11.225, -26.645) -> (-0.925, -26.645) projected
  line L3 (11.225, -12.495) -> (11.225, -26.645) projected
  line L4 (-0.925, -12.495) -> (11.225, -12.495) projected
  line L5 (-0.925, -17.0932) -> (-0.925, -12.495) projected
  spline S2 degree 5 poles (0.075, -16.0632) (-0.1182, -16.2756) (-0.315, -16.4848) (-0.5151, -16.6908) (-0.7185, -16.8936) (-0.925, -17.0932) knots 0 0 0 0 0 0 1 1 1 1 1 1 projected
  spline S3 degree 7 poles (0.075, -16.0632) (0.0824, -16.055) (0.1032, -16.0321) (0.1269, -16.006) (0.1481, -15.9825) (0.1654, -15.9632) (0.1818, -15.945) (0.446, -15.6493) (0.6834, -15.373) (0.9153, -15.0921) (1.1415, -14.8065) (1.3619, -14.5164) (1.5762, -14.2219) (1.7844, -13.9232) knots 0 0 0 0 0 0 0 0 0.081602 0.081602 0.081602 0.081602 0.081602 0.081602 1 1 1 1 1 1 1 1 projected
  spline S4 degree 2 poles (2.6048, -13.495) (2.3181, -13.495) (2.075, -13.6469) (1.9015, -13.7553) (1.7844, -13.9232) knots 0 0 0 0.578893 0.578893 1 1 1 weights 1 0.961275 1 0.979699 1 projected
  line L6 (8.225, -13.495) -> (2.6048, -13.495) projected
  line L7 (8.225, -13.495) -> (8.225, -25.645) projected
  line L8 (-0.925, -26.645) -> (-0.925, -12.495) projected
  line L9 (-0.925, -12.495) -> (11.225, -12.495) projected
  line L10 (-0.925, -26.645) -> (2.075, -26.645)
  line L11 (2.075, -26.645) -> (2.075, -12.495)
  line L12 (2.075, -12.495) -> (-0.925, -12.495)
  line L13 (-0.925, -12.495) -> (-0.925, -26.645)
  line L14 (-0.925, -17.0932) -> (-0.925, -25.7704) projected
  spline S5 degree 2 poles (-7.8131, -26.9469) (-3.9562, -26.0517) (-0.925, -25.7704) knots 0 0 0 1 1 1 projected
  spline S6 degree 6 poles (-9.8275, -33.5784) (-10.0654, -33.3246) (-10.2767, -33.0459) (-10.4584, -32.7459) (-10.6077, -32.4285) (-10.7227, -32.0982) (-10.8824, -31.4196) (-10.9267, -31.0712) (-10.9344, -30.7191) (-10.905, -30.3682) (-10.8393, -30.0232) (-10.6376, -29.3544) (-10.5018, -29.0305) (-10.3322, -28.7218) (-10.1313, -28.4327) (-9.9017, -28.1668) (-9.3916, -27.6877) (-9.1107, -27.4745) (-8.8081, -27.2915) (-8.4879, -27.1414) (-8.1547, -27.0262) (-7.8131, -26.9469) knots 0 0 0 0 0 0 0 0.249 0.249 0.249 0.249 0.249 0.499 0.499 0.499 0.499 0.499 0.749 0.749 0.749 0.749 0.749 1 1 1 1 1 1 1 projected
  spline S7 degree 6 poles (-9.7943, -22.7665) (-9.9651, -22.8392) (-10.1428, -22.9037) (-10.3268, -22.9589) (-10.5163, -23.0039) (-10.7102, -23.038) (-11.0425, -23.0759) (-11.1789, -23.086) (-11.3166, -23.0904) (-11.4552, -23.0892) (-11.5944, -23.0821) (-11.8312, -23.06) (-11.9289, -23.0479) (-12.0265, -23.033) (-12.1239, -23.0151) (-12.2209, -22.9943) (-12.5466, -22.9142) (-12.7731, -22.8412) (-12.9949, -22.7519) (-13.2103, -22.6466) (-13.4176, -22.526) (-13.8129, -22.2565) (-14.0009, -22.1075) (-14.1776, -21.9455) (-14.3418, -21.7716) (-14.4924, -21.5874) (-14.6859, -21.3135) (-14.7408, -21.2308) (-14.793, -21.1466) (-14.8425, -21.0612) (-14.8894, -20.9747) (-14.9965, -20.7623) (-15.0539, -20.6353) (-15.1057, -20.5068) (-15.1519, -20.3769) (-15.1924, -20.2463) (-15.2784, -19.9231) (-15.3175, -19.7301) (-15.3448, -19.5373) (-15.3606, -19.3459) (-15.3655, -19.1569) (-15.3601, -18.9713) knots 0 0 0 0 0 0 0 0.151603 0.151603 0.151603 0.151603 0.151603 0.255165 0.255165 0.255165 0.255165 0.255165 0.32775 0.32775 0.32775 0.32775 0.32775 0.5 0.5 0.5 0.5 0.5 0.67225 0.67225 0.67225 0.67225 0.67225 0.744835 0.744835 0.744835 0.744835 0.744835 0.848397 0.848397 0.848397 0.848397 0.848397 1 1 1 1 1 1 1 projected
  spline S8 degree 2 poles (-0.925, -17.0932) (-4.4331, -20.4829) (-9.7943, -22.7665) knots 0 0 0 1 1 1 projected
  arc A0 (-15.3601, -18.9713) -> (-9.8275, -33.5784) centre (5.1314, -19.5612) ccw projected
  point P0 (0, 0)
  point P1 (-0.925, -25.7704)
  point P2 (-0.925, -25.7704)
  point P3 (2.075, -13.6469)
  dimension "d62" = 3
  constraints: 8 end point, 2 parallel, 1 horizontal, 1 perpendicular, 1 point on line, 9 other
  measures "d62" distance of L12.end L11.end
extrude "Wyciągnięcie proste13" add sketch "Szkic13" along normal mid plane 1 contours S5 S6 A0 S7 S8 L8
extrude "Wyciągnięcie proste14" add sketch "Szkic13" against normal up to surface (0.5 mm away) contours S0 S1 L8 S2 S3 S4 L11 | S4 S3 S2 L5 L4 L11
extrude "Wyciągnięcie proste15" add sketch "Szkic13" against normal blind 5 contours S0 S1 L8 S2 S3 S4 L11 | S5 S6 A0 S7 S8 L8
sketch "Szkic14" plane through (0, 0, 4.7) normal (0, 0, 1) x (1, 0, 0)
  line L0 (-0.925, -26.645) -> (-0.925, -12.495) projected
  line L1 (11.225, -26.645) -> (-0.925, -26.645) projected
  line L2 (11.225, -12.495) -> (11.225, -26.645) projected
  line L3 (-0.925, -12.495) -> (11.225, -12.495) projected
  line L4 (2.075, -25.645) -> (2.075, -13.6469) projected
  spline S0 degree 2 poles (2.6048, -13.495) (2.3181, -13.495) (2.075, -13.6469) knots 0 0 0 1 1 1 weights 1 0.961275 1 projected
  line L5 (8.225, -13.495) -> (2.6048, -13.495) projected
  line L6 (8.225, -13.495) -> (8.225, -25.645) projected
  line L7 (2.075, -25.645) -> (8.225, -25.645) projected
  point P0 (0, 0)
  constraints: 1 other
extrude "Wyciągnięcie proste16" cut sketch "Szkic14" against normal blind 2
